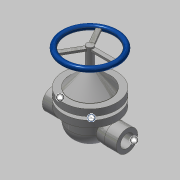
# Autodesk Inventor part: MANUEL BUTTWELD DIAFRAGM VALVE DN32
Saved by Autodesk Inventor 2017 (Build 210142000, 142)
## iProperties
Category: Piping Part
Company: Demarec
Created: 2012-12-20
Part Number: MANUEL BUTTWELD DIAFRAGM VALVE DN32
Material: 304L
Document SubType Name: Modeling
Designer: Marc Crauwels
Density: 8 g/cm^3
Mass: 658107 g
Surface Area: 21375.3 cm^2
Volume: 83622.3 cm^3
Appearance: Steel
Catalog Web Link: http://www.pocketbrewery.com
Author: Marc Crauwels
Title: Carbon Steel Globe Valve PN16
Comments: iPart CS GlbVlvPN16
Autodesk Inventor part; units mm, degrees
ref_plane "YZ Plane" through (0, 0, 0) normal (1, 0, 0) x (0, 1, 0)
ref_plane "XZ Plane" through (0, 0, 0) normal (0, 1, 0) x (-1, 0, 0)
ref_plane "XY Plane" through (0, 0, 0) normal (0, 0, 1) x (1, 0, 0)
sketch "Sketch1" plane through (0, 0, 0) normal (1, 0, 0) x (0, 1, 0)
  line L0 (74, 16) -> (88, 16)
  line L1 (88, 16) -> (88, 70)
  line L2 (88, 70) -> (74, 70)
  line L3 (74, 70) -> (74, 16)
  line L4 (88, 16) -> (90, 16)
  line L5 (90, 16) -> (90, 36)
  line L6 (90, 36) -> (88, 36)
  line L7 (88, 36) -> (88, 16)
  line L8 (-90, 0) -> (90, 0) construction
  line L9 (90, 0) -> (74, 0) construction
  line L10 (0, 0) -> (0, 157) construction
  line L11 (-90, 0) -> (-74, 0) construction
  line L12 (0, 0) -> (-8.4, 0)
  line L13 (-8.4, 0) -> (-8.4, 157)
  line L14 (-8.4, 157) -> (0, 157)
  line L15 (0, 157) -> (0, 0)
  line L16 (-8.4, 153.2) -> (-63, 153.2)
  line L17 (-63, 153.2) -> (-63, 148.2)
  line L18 (-63, 148.2) -> (-8.4, 148.2)
  line L19 (-8.4, 148.2) -> (-8.4, 153.2)
  circle A0 centre (-63, 150.7) radius 6.3
  line L20 (0, 0) -> (0, -33)
  line L21 (49, 0) -> (49, 28)
  line L22 (49, 28) -> (65, 28)
  line L23 (65, 28) -> (65, 44)
  line L24 (65, 44) -> (49, 44)
  line L25 (49, 44) -> (49, 52)
  line L26 (49, 52) -> (65, 52)
  line L27 (65, 52) -> (65, 68)
  line L28 (65, 68) -> (49, 68)
  line L29 (49, 68) -> (49, 68.75)
  line L30 (49, 68.75) -> (0, 117.75)
  line L31 (0, 117.75) -> (0, 0)
  line L32 (0, -33) -> (16, -33)
  arc A1 (16, -33) -> (49, 0) centre (16, 0) ccw
  line L33 (88, 36) -> (65, 36) construction
  dimension "Lenght" = 180
  dimension "DN" = 32
  dimension "FlgDia" = 140
  dimension "FlgThck" = 16
  dimension "GsktFace" = 72
  dimension "d48" = 8.4
  dimension "d49" = 12.6
  dimension "d50" = 5
  dimension "d51" = 63
  dimension "Face" = 2
  dimension "d79" = 157
  dimension "d101" = 16
  dimension "d102" = 8
  dimension "d104" = 130
  dimension "d105" = 45
  dimension "d108" = 117.75
  constraints: 68 end point, 13 perpendicular, 11 point on line, 8 parallel, 5 horizontal, 4 collinear, 4 equal length, 3 midpoint, 3 tangent, 2 centre point, 2 coincident, 2 point on circle, 2 vertical
  measures "Lenght" distance of L8.start L8.end
  measures "DN" diameter of L0 L8
  measures "FlgDia" diameter of L2 L8
  measures "FlgThck" distance between parallel lines of L3 L5
  measures "GsktFace" diameter of L5.end L8
  measures "d48" distance of L13.end L14.end
  measures "d49" diameter of A0
  measures "d50" distance of L16.end L17.end
  measures "d51" distance from line of A0.centre L10
  measures "Face" distance of L5.end L6.end
  measures "d79" distance of L12.end L13.end
  measures "d101" distance of L22.end L23.end
  measures "d102" distance of L24.end L25.end
  measures "d104" diameter of L23 L31
  measures "d105" angle of L31 L30
  measures "d108" distance from line of L30.end L12
revolve "Revolution1" add sketch "Sketch1" angle 360 about axis through (0, -90, 0) along (0, 1, 0) contours L3 L2 L1 L0 | L1 L6 L5 L4
sketch "Sketch14" plane through (0, 74, 0) normal (0, -1, 0) x (-1, 0, 0)
  circle A0 centre (0, 0) radius 16 projected
  circle A1 centre (0, 0) radius 26
  dimension "d54" = 10
  dimension "d84" = 52
  constraints: 1 centre point
  measures "d54" radial gap between concentric circles of A1 A0
  measures "d84" diameter of A1
sketch "Sketch20" plane through (0, 0, 0) normal (1, 0, 0) x (0, 1, 0)
  line L0 (74, 36) -> (74, -36)
  line L1 (74, 0) -> (61, 0)
  arc A0 (0, 61) -> (61, 0) centre (61, 61) ccw
  line L2 (0, 61) -> (0, 66)
  line L3 (74, -70) -> (74, 70) projected
  line L4 (90, -36) -> (90, 36) projected
  point P0 (0, 0)
  point P1 (0, 0)
  dimension "d80" = 25
  dimension "d81" = 5
  constraints: 6 end point, 2 point on circle, 2 point on line, 2 tangent, 1 centre point, 1 coincident, 1 collinear, 1 horizontal, 1 midpoint, 1 parallel, 1 perpendicular
  measures "d80" vertical distance of L0.start L2.start
  measures "d81" distance of L2.start L2.end
sweep "Sweep4" add profiles "Sketch14" path "Sketch20" path curves L1 A0 L2
mirror "Mirror2" about plane through (0, 0, 0) normal (0, 1, 0) of "Revolution1", "Sweep4"
revolve "Revolution3" add sketch "Sketch1" angle 360 about axis through (0, 0, 0) along (0, 0, 1) contours L12 L13 L14 L15 | L18 A0 L16 L13 | A0 L16 L17 L18 | L18 L17 L16 A0
sketch "Sketch16" plane through (0, 0, 153.2) normal (0, 0, 1) x (1, 0, 0)
  line L0 (0, 0) -> (0, 112.0641) construction
  line L1 (0, 0) -> (89.1399, 51.465) construction
  line L2 (0, 0) -> (-84.4387, 48.7507) construction
  line L3 (-46.839, 32.8622) -> (-3.2997, 7.7248)
  line L4 (46.839, 32.8622) -> (3.2997, 7.7248)
  circle A0 centre (0, 0) radius 8.4 projected
  circle A1 centre (0, 0) radius 57.2173 projected
  arc A2 (3.2997, 7.7248) -> (-3.2997, 7.7248) centre (0, 0) ccw
  arc A3 (46.839, 32.8622) -> (-46.839, 32.8622) centre (0, 0) ccw
  dimension "d61" = 120
  dimension "d62" = 60
  dimension "d63" = 5.04
  dimension "d64" = 5.04
  constraints: 10 end point, 8 point on circle, 2 centre point, 2 coincident, 2 concentric, 2 parallel, 1 vertical
  measures "d61" angle of L1 L2
  measures "d62" angle of L0 L1
  measures "d63" distance between parallel lines of L3 L2
  measures "d64" distance between parallel lines of L1 L4
extrude "Extrusion6" cut sketch "Sketch16" against normal blind 5 contours A1 L4 A0 L3 picked at (-30.1888, 27.0255)
pattern_circular "Circular Pattern3" count 3 over 360 about axis through (0, 0, 155.1) along (0, 0, 1) of "Extrusion6"
revolve "Revolution5" add sketch "Sketch1" angle 360 about axis through (0, 0, 117.75) along (0, 0, -1) contours L15 L30 L29 L28 L27 L26 L25 L24 L23 L22 L21 A1 L32 L20
sketch "Sketch25" plane through (0, 90, 0) normal (0, 1, 0) x (1, 0, 0)
  circle A0 centre (0, 0) radius 26 projected
  circle A1 centre (0, 0) radius 70 projected
extrude "Extrusion11" cut sketch "Sketch25" against normal up to surface (16 mm away)
mirror "Mirror3" about plane through (0, 0, 0) normal (0, 1, 0) of "Extrusion11"
equation "\"d51\" = 0.5 * WhlDia"
equation "\"WhlDia\" = 126"
equation "\"Height\" = 207"
body "Solid1"
